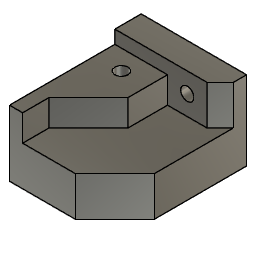
robocon_cad1 v1 (Autodesk Fusion 360 design; units mm, degrees)
Autodesk Fusion 360 part; units mm, degrees
sketch "Sketch1" plane through (0, 0, 0) normal (0, 1, 0) x (1, 0, 0)
  line L0 (8, 6) -> (-8, 6)
  line L1 (-8, 6) -> (-8, -6)
  line L2 (-8, -6) -> (8, -6)
  line L3 (8, -6) -> (8, 6)
  line L4 (8, 6) -> (-8, -6) construction
  line L5 (-8, 6) -> (8, -6) construction
  dimension "d1" = 16
  dimension "d2" = 12
  constraint horizontal L0
  constraint perpendicular L0 L1
  constraint parallel L0 L2
  constraint parallel L1 L3
  constraint coincident L4 origin
  constraint coincident L5 origin
  measures "d1" distance of L1.end L2.end
  measures "d2" distance of L0.end L1.end
extrude "Extrude1" add sketch "Sketch1" against normal blind 2
sketch "Sketch2" plane through (0, -2, 0) normal (0, -1, 0) x (1, 0, 0)
  line L0 (8, -6) -> (8, 6)
  line L1 (8, 6) -> (-8, 6)
  line L2 (-8, 6) -> (-8, -6)
  line L3 (-8, -6) -> (8, -6)
  line L4 (-8, 6) -> (6, 6)
  line L5 (6, 6) -> (6, 0)
  line L6 (6, 0) -> (-8, 0)
  line L7 (-8, 0) -> (-8, 6)
  dimension "d5" = 14
  constraint horizontal L4
  constraint vertical L5
  constraint horizontal L6
  constraint vertical L7
  constraint coincident L1.end L2.start
  measures "d5" distance of L1.end L4.end
extrude "Extrude2" add sketch "Sketch2" along normal blind 2 contours L1 L2 L4 L5 L6 L7
sketch "Sketch3" plane through (0, 0, 6) normal (0, 0, 1) x (-1, 0, 0)
  line L0 (-8, 0) -> (8, 0)
  line L1 (8, 0) -> (8, 4)
  line L2 (8, 4) -> (-6, 4)
  line L3 (-6, 4) -> (-6, 2)
  line L4 (-6, 2) -> (-8, 2)
  line L5 (-8, 2) -> (-8, 0)
  line L6 (-6, 4) -> (-8, 2)
  constraint coincident L2.end L3.start
  constraint coincident L4.end L5.start
extrude "Extrude3" add sketch "Sketch3" against normal blind 6 contours L3 L4 L6
sketch "Sketch4" plane through (0, -4, 0) normal (0, -1, 0) x (1, 0, 0)
  line L0 (-8, 0) -> (6, 0)
  line L1 (6, 0) -> (6, 6)
  line L2 (6, 6) -> (-8, 6)
  line L3 (-8, 6) -> (-8, 0)
  line L4 (-8, 0) -> (0, 0)
  line L5 (0, 0) -> (0, 4)
  line L6 (0, 4) -> (-8, 4)
  line L7 (-8, 4) -> (-8, 0)
  dimension "d10" = 8
  dimension "d11" = 4
  constraint horizontal L4
  constraint vertical L5
  constraint horizontal L6
  constraint vertical L7
  constraint coincident L0.start L3.end
  measures "d10" distance of L0.start L4.end
  measures "d11" distance of L0.start L6.end
extrude "Extrude4" add sketch "Sketch4" along normal blind 6 contours L0 L3 L4 L5 L6 L7
sketch "Sketch5" plane through (0, -10, 0) normal (0, -1, 0) x (1, 0, 0)
  line L0 (-8, 4) -> (-8, 0)
  line L1 (-8, 0) -> (0, 0)
  line L2 (0, 0) -> (0, 4)
  line L3 (0, 4) -> (-8, 4)
  line L4 (-8, 4) -> (-6, 4)
  line L5 (-6, 4) -> (-6, 0)
  line L6 (-6, 0) -> (-8, 0)
  line L7 (-8, 0) -> (-8, 4)
  dimension "d14" = 2
  dimension "d15" = 4
  constraint horizontal L4
  constraint vertical L5
  constraint horizontal L6
  constraint vertical L7
  constraint coincident L0.start L3.end
  measures "d14" distance of L0.start L4.end
  measures "d15" distance of L0.start L0.end
extrude "Extrude5" add sketch "Sketch5" along normal blind 10 contours L0 L1 L3 L4 L5 L6 L7
sketch "Sketch6" plane through (0, 0, 4) normal (0, 0, 1) x (-1, 0, 0)
  line L0 (0, 4) -> (8, 4)
  line L1 (8, 4) -> (8, 20)
  line L2 (8, 20) -> (6, 20)
  line L3 (6, 20) -> (6, 10)
  line L4 (6, 10) -> (0, 10)
  line L5 (0, 10) -> (0, 4)
  line L6 (6, 10) -> (6, 16) construction
  line L7 (6, 16) -> (0, 10)
  dimension "d18" = 6
  constraint coincident L3.end L4.start
  constraint perpendicular L4 L6
  constraint coincident L4.end L5.start
  measures "d18" distance of L3.end L6.end
extrude "Extrude6" add sketch "Sketch6" against normal blind 4 contours L3 L4 L7
sketch "Sketch7" plane through (0, -2, 0) normal (0, -1, 0) x (1, 0, 0)
  line L0 (8, 0) -> (-8, 0)
  line L1 (-8, 0) -> (-8, -6)
  line L2 (-8, -6) -> (8, -6)
  line L3 (8, -6) -> (8, 0)
  line L4 (-8, 0) -> (8, 0)
  line L5 (8, 0) -> (8, -6)
  line L6 (8, -6) -> (-8, -6)
  line L7 (-8, -6) -> (-8, 0)
  constraint horizontal L4
  constraint vertical L5
  constraint horizontal L6
  constraint vertical L7
  constraint coincident L2.end L3.start
  constraint coincident L0.end L1.start
extrude "Extrude7" add sketch "Sketch7" along normal blind 12
sketch "Sketch8" plane through (0, -14, 0) normal (0, -1, 0) x (1, 0, 0)
  line L0 (-8, -6) -> (8, -6)
  line L1 (8, -6) -> (8, 0)
  line L2 (8, 0) -> (-4, 0)
  line L3 (-4, 0) -> (-8, 0)
  line L4 (-8, 0) -> (-8, -6)
  line L5 (-8, 0) -> (2, 0)
  line L6 (2, 0) -> (2, -6)
  line L7 (2, -6) -> (-8, -6)
  line L8 (-8, -6) -> (-8, 0)
  dimension "d23" = 10
  dimension "d24" = 6
  constraint horizontal L5
  constraint vertical L6
  constraint horizontal L7
  constraint vertical L8
  constraint coincident L3.end L4.start
  measures "d23" distance of L3.end L5.end
  measures "d24" distance of L3.end L0.start
extrude "Extrude8" add sketch "Sketch8" along normal blind 6 contours L0 L2 L3 L4 L5 L6 L7 L8
sketch "Sketch9" plane through (0, 0, 0) normal (0, 0, 1) x (-1, 0, 0)
  line L0 (0, 10) -> (6, 16)
  line L1 (6, 16) -> (6, 20)
  line L2 (6, 20) -> (-2, 20)
  line L3 (-2, 20) -> (-2, 14)
  line L4 (-2, 14) -> (-8, 14)
  line L5 (-8, 14) -> (-8, 2)
  line L6 (-8, 2) -> (-6, 4)
  line L7 (-6, 4) -> (0, 4)
  line L8 (0, 4) -> (0, 10)
  line L9 (-2, 20) -> (-8, 14)
  constraint coincident L2.end L3.start
  constraint coincident L4.end L5.start
extrude "Extrude9" add sketch "Sketch9" against normal blind 6 contours L3 L4 L9
sketch "Sketch10" plane through (0, -4, 0) normal (0, -1, 0) x (1, 0, 0)
  line L0 (0, 4) -> (0, 0)
  line L1 (0, 0) -> (6, 0)
  line L2 (6, 0) -> (6, 6)
  line L3 (6, 6) -> (-8, 6)
  line L4 (-8, 6) -> (-8, 4)
  line L5 (-8, 4) -> (0, 4)
  circle A0 centre (3, 3) radius 1
  dimension "d30" = 2
  measures "d30" diameter of A0
extrude "Extrude10" cut sketch "Sketch10" against normal up to surface (4 mm away) contours A0
sketch "Sketch11" plane through (0, 0, 4) normal (0, 0, 1) x (-1, 0, 0)
  line L0 (0, 4) -> (8, 4)
  line L1 (8, 4) -> (8, 20)
  line L2 (8, 20) -> (6, 20)
  line L3 (6, 20) -> (6, 16)
  line L4 (6, 16) -> (0, 10)
  line L5 (0, 10) -> (0, 4)
  circle A0 centre (4, 7) radius 1
  dimension "d33" = 2
  measures "d33" diameter of A0
extrude "Extrude11" cut sketch "Sketch11" against normal up to surface (10 mm away) contours A0
